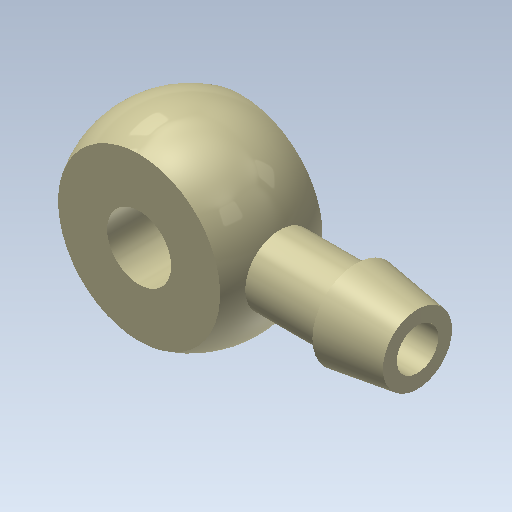
# Autodesk Inventor part: Fuel Intake
Saved by Autodesk Inventor 2020 (Build 240152000, 152)
## iProperties
Created: 2012-08-08
Part Number: Fuel Intake
Material: Nylon, molybdenum disulphide
Document SubType Name: Modeling
Designer: John
Mass: 0.36445 g
Surface Area: 4.27579 cm^2
Volume: 0.322522 cm^3
Density: 1.13 g/cm^3
Appearance: Nylon 6
Author: John
Autodesk Inventor part; units mm, degrees
note: some values were not read from the file. Chosen so that the rebuilt part matches the saved one: direction of "Hole2".
ref_plane "YZ Plane" through (0, 0, 0) normal (1, 0, 0) x (0, 1, 0)
ref_plane "XZ Plane" through (0, 0, 0) normal (0, 1, 0) x (-1, 0, 0)
ref_plane "XY Plane" through (0, 0, 0) normal (0, 0, 1) x (1, 0, 0)
sketch "Sketch2" plane through (0, 0, 0) normal (0, 0, 1) x (1, 0, 0)
  circle A0 centre (0, 0) radius 4.7498
  line L0 (4.7498, 0) -> (-4.7498, 0)
  dimension "d1" = 4.7498
  constraints: 2 end point, 2 point on circle, 1 centre point, 1 coincident, 1 midpoint
  measures "d1" radius of A0
revolve "Revolution1" add sketch "Sketch2" angle 360 about axis through (4.7498, 0, 0) along (-1, 0, 0) picked at (-0.543, 3.0005) contours L0 A0
sketch "Sketch3" plane through (0, 0, 0) normal (0, 1, 0) x (-1, 0, 0)
  arc A0 (0, 4.7498) -> (0, -4.7498) centre (0, 0) ccw projected
  arc A1 (0, -4.7498) -> (0, 4.7498) centre (0, 0) ccw projected
  line L0 (-4.7498, 2.54) -> (4.7498, 2.54)
  line L1 (4.7498, 2.54) -> (4.7498, -2.54)
  line L2 (4.7498, -2.54) -> (-4.7498, -2.54)
  line L3 (-4.7498, -2.54) -> (-4.7498, 2.54)
  line L4 (0, 0) -> (0, 2.54)
  line L5 (-4.7498, 2.54) -> (4.7498, 2.54)
  line L6 (4.7498, 2.54) -> (4.7498, 4.7498)
  line L7 (4.7498, 4.7498) -> (-4.7498, 4.7498)
  line L8 (-4.7498, 4.7498) -> (-4.7498, 2.54)
  line L9 (-4.7498, -2.54) -> (4.7498, -2.54)
  line L10 (4.7498, -2.54) -> (4.7498, -4.7498)
  line L11 (4.7498, -4.7498) -> (-4.7498, -4.7498)
  line L12 (-4.7498, -4.7498) -> (-4.7498, -2.54)
  dimension "d3" = 5.08
  dimension "d5" = 2.54
  constraints: 26 end point, 6 parallel, 3 horizontal, 3 perpendicular, 3 tangent, 2 collinear, 1 midpoint, 1 vertical
  measures "d3" distance of L2.end L0.start
  measures "d5" distance of L4.start L4.end
extrude "Extrusion1" cut sketch "Sketch3" along normal mid plane 25.4 contours A1 L0 A0 | L7 L6 L0 A1 | A0 L0 L8 L7 | L2 A1 A0 | A0 L11 L12 L2 | L2 L10 L11 A1
sketch "Sketch5" plane through (0, 0, 0) normal (0, 1, 0) x (-1, 0, 0)
  line L0 (4.0136, -2.54) -> (-4.0136, -2.54) projected
  arc A0 (-4.0136, 2.54) -> (-4.0136, -2.54) centre (0, 0) ccw projected
  line L1 (-4.0136, 2.54) -> (4.0136, 2.54) projected
  arc A1 (4.0136, -2.54) -> (4.0136, 2.54) centre (0, 0) ccw projected
  line L2 (0, 0) -> (-18.5035, 0)
  line L3 (-11.2518, 0) -> (-11.2518, 1.7145)
  line L4 (-11.2518, 1.7145) -> (-8.2038, 2.159)
  line L5 (-8.2038, 2.159) -> (-8.2038, 1.7145)
  line L6 (-8.2038, 1.7145) -> (-4.4296, 1.7145)
  line L7 (-4.4296, 1.7145) -> (-4.4296, 0)
  line L8 (-11.2518, 0) -> (-4.4296, 0)
  dimension "d12" = 4.0136
  dimension "d15" = 3.429
  dimension "d16" = 4.318
  dimension "d17" = 15.2654
  dimension "d18" = 12.2174
  constraints: 14 end point, 3 perpendicular, 2 parallel, 2 point on line, 1 collinear, 1 horizontal alignment, 1 point on circle
  measures "d12" horizontal distance of point (0, 0) L0.start
  measures "d15" diameter of L3.end L2
  measures "d16" diameter of L4.end L2
  measures "d17" distance from line of L0.start L3
  measures "d18" distance from line of L0.start L5
revolve "Revolution2" add sketch "Sketch5" angle 360 about axis through (0, 0, 0) along (1, 0, 0) contours L2 L3 L4 L5 L6 A0 | A0 L7 L2
sketch "Sketch6" plane through (0, 0, 2.54) normal (0, 0, 1) x (1, 0, 0)
  circle A0 centre (0, 0) radius 4.0136 projected
hole "Hole1" at (0, 0, 2.54) direction (0, 0, -1) diameter 3.175 end through all
sketch "Sketch7" plane through (11.2518, 0, 0) normal (1, 0, 0) x (0, 0, -1)
  circle A0 centre (0, 0) radius 1.7145 projected
hole "Hole2" at (11.2518, 0, 0) direction (-1, 0, 0) diameter 2.0574 end up to surface clearance for "Flat Head Machine Screw (82)" size "#1" standard "Ansi Unified Screw Threads"
equation "\"d5\" = 0.5 * d3"
body "Solid1"
